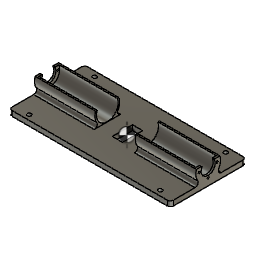
Bottenplatta v15 (Autodesk Fusion 360 design; units mm, degrees)
Autodesk Fusion 360 part; units mm, degrees
note: some values were not read from the file. Chosen so that the rebuilt part matches the saved one: add or cut; which face or edge a step refers to; which sketch regions a step uses.
sketch "Sketch1" plane through (0, 0, 0) normal (0, 0, 1) x (1, 0, 0)
  line L0 (-47, 8.9127) -> (107, 8.9127)
  line L1 (110, 11.9127) -> (110, 80.9127)
  line L2 (107, 83.9127) -> (-47, 83.9127)
  line L3 (-50, 80.9127) -> (-50, 11.9127)
  circle A0 centre (-35, 78.9127) radius 2
  line L4 (-70.7601, 46.4127) -> (89.2399, 46.4127)
  line L5 (30, -13.009) -> (30, 54.6952)
  circle A1 centre (95, 78.9127) radius 2
  circle A2 centre (-35, 13.9127) radius 2
  circle A3 centre (95, 13.9127) radius 2
  arc A4 (-47, 83.9127) -> (-50, 80.9127) centre (-47, 80.9127) ccw
  arc A5 (110, 80.9127) -> (107, 83.9127) centre (107, 80.9127) ccw
  arc A6 (107, 8.9127) -> (110, 11.9127) centre (107, 11.9127) ccw
  arc A7 (-50, 11.9127) -> (-47, 8.9127) centre (-47, 11.9127) ccw
  line L6 (35, 36.4127) -> (25, 36.4127)
  line L7 (25, 36.4127) -> (25, 56.4127)
  line L8 (25, 56.4127) -> (35, 56.4127)
  line L9 (35, 56.4127) -> (35, 36.4127)
  point P0 (110, 8.9127)
  point P1 (110, 83.9127)
  point P2 (-50, 83.9127)
  dimension "d3" = 4
  dimension "d4" = 15
  dimension "d5" = 5
  dimension "d6" = 75
  dimension "d7" = 160
  dimension "d9" = 75
  dimension "d12" = 3
  dimension "d13" = 160
  dimension "d48" = 50
  dimension "d57" = 20
  dimension "d58" = 10
  dimension "d59" = 27.5
  dimension "d60" = 75
  constraint horizontal L0
  constraint vertical L1
  constraint horizontal L2
  constraint vertical L3
  constraint perpendicular L1 L4
  constraint perpendicular L2 L5
  constraint symmetric A0 L5 A1
  constraint symmetric A0 L4 A2
  constraint symmetric L4 A1 A3
  constraint coincident P2 L2
  constraint coincident P2 L3
  constraint tangent L2 A4
  constraint tangent L3 A4
  constraint coincident P1 L1
  constraint coincident P1 L2
  constraint tangent L1 A5
  constraint tangent L2 A5
  constraint equal A4 A5
  constraint coincident P0 L0
  constraint coincident P0 L1
  constraint tangent L0 A6
  constraint tangent L1 A6
  constraint equal A4 A6
  constraint tangent L0 A7
  constraint tangent L3 A7
  constraint equal A4 A7
  constraint horizontal L6
  constraint vertical L7
  constraint horizontal L8
  constraint vertical L9
  measures "d3" diameter of A0
  measures "d4" distance of L3 A0.centre
  measures "d5" distance of L2 A0.centre
  measures "d6" distance of P0 P1
  measures "d7" distance of P1 P2
  measures "d12" radius of A4
  measures "d48" distance of origin L3
  measures "d57" distance of L6.start L8.end
  measures "d58" distance of L6.start L6.end
  measures "d59" distance of L0 L6
  measures "d60" distance of L1 L9
extrude "Extrude1" add sketch "Sketch1" along normal blind 3 contours L0 L3 L4 L5 A7 L6 L7 | L0 L1 L2 L3 L4 L5 A4 A5 A6 L6 L7 L8 L9
sketch "Sketch2" plane through (0, 0, 0) normal (0, 0, -1) x (1, 0, 0)
  circle A0 centre (95, -78.9127) radius 2
  circle A1 centre (-35, -13.9127) radius 2
  circle A2 centre (95, -13.9127) radius 2
  circle A3 centre (-35, -78.9127) radius 2
  arc A4 (-47, -8.9127) -> (-50, -11.9127) centre (-47, -11.9127) ccw
  line L0 (-50, -11.9127) -> (-50, -80.9127)
  arc A5 (-50, -80.9127) -> (-47, -83.9127) centre (-47, -80.9127) ccw
  line L1 (-47, -83.9127) -> (107, -83.9127)
  arc A6 (107, -83.9127) -> (110, -80.9127) centre (107, -80.9127) ccw
  line L2 (110, -80.9127) -> (110, -11.9127)
  arc A7 (110, -11.9127) -> (107, -8.9127) centre (107, -11.9127) ccw
  line L3 (107, -8.9127) -> (-47, -8.9127)
  line L4 (35, -56.4127) -> (25, -56.4127)
  line L5 (25, -56.4127) -> (25, -36.4127)
  line L6 (25, -36.4127) -> (35, -36.4127)
  line L7 (35, -36.4127) -> (35, -56.4127)
sketch "Sketch3" plane through (-50, 0, 0) normal (-1, 0, 0) x (0, -1, 0)
  line L0 (-80.9127, 0) -> (-11.9127, 0)
  line L1 (-11.9127, 0) -> (-11.9127, 3)
  line L2 (-11.9127, 3) -> (-80.9127, 3)
  line L3 (-80.9127, 3) -> (-80.9127, 0)
  circle A0 centre (-46.4127, 14) radius 10.8
  line L4 (-11.9127, 0) -> (-80.9127, 0)
  circle A1 centre (-46.4127, 14) radius 12.3
  line L5 (-33, 21) -> (-5, 21)
  line L6 (-83.9127, 0) -> (-83.9127, 3)
  line L7 (-8.9127, 0) -> (-8.9127, 3)
  dimension "d14" = 21.6
  dimension "d15" = 14
  dimension "d16" = 1.5
  dimension "d33" = 75
  dimension "d34" = 37.5
  constraint horizontal L5
  measures "d14" diameter of A0
  measures "d15" distance of A0.centre L4
  measures "d33" distance of L6 L7
  measures "d34" distance of A0.centre L7
sketch "Sketch4" plane through (110, 0, 0) normal (1, 0, 0) x (0, 1, 0)
  line L0 (11.9127, 0) -> (80.9127, 0)
  line L1 (80.9127, 0) -> (80.9127, 3)
  line L2 (80.9127, 3) -> (11.9127, 3)
  line L3 (11.9127, 3) -> (11.9127, 0)
  circle A0 centre (46.4127, 14) radius 10.8
  line L4 (33, 21) -> (5, 21)
  circle A1 centre (46.4127, 14) radius 12.3
extrude "Extrude2" add sketch "Sketch4" against normal blind 60 contours L2 A1 picked at (35.797, 8.8983)
extrude "Extrude3" add sketch "Sketch3" against normal blind 60 contours L2 A1 picked at (-57.0284, 8.8983)
sketch "Sketch5" plane through (110, 0, 0) normal (1, 0, 0) x (0, 1, 0)
  circle A0 centre (46.4127, 14) radius 10.8
  line L0 (11.9127, 0) -> (80.9127, 0)
  line L1 (80.9127, 0) -> (80.9127, 3)
  line L2 (80.9127, 3) -> (51.9163, 3)
  arc A1 (51.9163, 3) -> (40.9091, 3) centre (46.4127, 14) ccw
  line L3 (40.9091, 3) -> (11.9127, 3)
  line L4 (11.9127, 3) -> (11.9127, 0)
  circle A2 centre (37.4127, 14) radius 1
  circle A3 centre (46.4127, 5) radius 1
  circle A4 centre (55.4127, 14) radius 1
  circle A5 centre (46.4127, 23) radius 1
  dimension "d23" = 2
  dimension "d24" = 9
  dimension "d26" = 360
  constraint horizontal A2.centre A4.centre
  measures "d23" diameter of A2
  measures "d24" distance of A0.centre A2.centre
extrude "Extrude4" add sketch "Sketch5" against normal blind 2 contours A0 | L0 L1 L2 A1 L3 L4
sketch "Sketch6" plane through (110, 0, 0) normal (1, 0, 0) x (0, 1, 0)
  circle A0 centre (37.4127, 14) radius 1
  circle A1 centre (46.4127, 5) radius 1
  circle A2 centre (55.4127, 14) radius 1
  circle A3 centre (46.4127, 23) radius 1
  line L0 (11.9127, 0) -> (80.9127, 0)
  line L1 (80.9127, 0) -> (80.9127, 3)
  line L2 (80.9127, 3) -> (51.9163, 3)
  arc A4 (51.9163, 3) -> (40.9091, 3) centre (46.4127, 14) ccw
  line L3 (40.9091, 3) -> (11.9127, 3)
  line L4 (11.9127, 3) -> (11.9127, 0)
  circle A5 centre (46.4127, 14) radius 7
  line L5 (46.4127, 14) -> (53.2094, 20.7967)
  line L6 (46.4127, 14) -> (51.6312, 14) construction
  dimension "d29" = 14
  dimension "d42" = 45
  constraint concentric A4 A5
  constraint horizontal L6
  constraint coincident A4.centre A5.centre
  measures "d29" diameter of A5
  measures "d42" angle of L5 L6
extrude "Extrude5" cut sketch "Sketch6" against normal blind 2 contours A5
sketch "Sketch7" plane through (-50, 0, 0) normal (-1, 0, 0) x (0, -1, 0)
  circle A0 centre (-46.4127, 14) radius 10.8
  line L0 (-80.9127, 0) -> (-11.9127, 0)
  line L1 (-11.9127, 0) -> (-11.9127, 3)
  line L2 (-11.9127, 3) -> (-40.9091, 3)
  arc A1 (-40.9091, 3) -> (-51.9163, 3) centre (-46.4127, 14) ccw
  line L3 (-51.9163, 3) -> (-80.9127, 3)
  line L4 (-80.9127, 3) -> (-80.9127, 0)
  line L5 (-70, 18) -> (-12.2133, 18)
  dimension "d37" = 15
  constraint horizontal L5
  measures "d37" distance of L2 L5
extrude "Extrude6" cut sketch "Sketch7" against normal through all contours A0 L5 | A0 A1 L5 picked at (-48.2013, 22.18)
fillet "Fillet2" radius 3 6 edges at (80, 40.9091, 3) (-20, 51.9163, 3) (-20, 51.9163, 3) (-20, 40.9091, 3) (80, 40.9091, 3) (80, 51.9163, 3)
sketch "Sketch8" plane through (-50, 0, 0) normal (-1, 0, 0) x (0, -1, 0)
  line L0 (-34.7813, 18) -> (-36.3808, 18)
  arc A0 (-56.4447, 18) -> (-36.3808, 18) centre (-46.4127, 14) ccw
  line L1 (-56.4447, 18) -> (-58.0441, 18)
  arc A1 (-58.0441, 18) -> (-56.8973, 7.5686) centre (-46.4127, 14) ccw
  arc A2 (-59.4546, 3) -> (-56.8973, 7.5686) centre (-59.4546, 6) ccw
  line L2 (-59.4546, 3) -> (-80.9127, 3)
  line L3 (-80.9127, 3) -> (-80.9127, 0)
  line L4 (-80.9127, 0) -> (-11.9127, 0)
  line L5 (-11.9127, 0) -> (-11.9127, 3)
  line L6 (-11.9127, 3) -> (-33.3709, 3)
  arc A3 (-35.9281, 7.5686) -> (-33.3709, 3) centre (-33.3709, 6) ccw
  arc A4 (-35.9281, 7.5686) -> (-34.7813, 18) centre (-46.4127, 14) ccw
  circle A5 centre (-37.4127, 14) radius 1
  circle A6 centre (-46.4127, 5) radius 1
  circle A7 centre (-55.4127, 14) radius 1
  line L7 (-36.3808, 18) -> (-40.6681, 18)
  arc A8 (-52.1573, 18) -> (-40.6681, 18) centre (-46.4127, 14) ccw
  line L8 (-52.1573, 18) -> (-56.4447, 18)
  arc A9 (-56.4447, 18) -> (-36.3808, 18) centre (-46.4127, 14) ccw
extrude "Extrude7" cut sketch "Sketch8" against normal blind 2 contours A0 L7 A8 L8 A9
fillet "Fillet3" radius 0.5 2 edges at (109, 52.1573, 18) (109, 40.6681, 18)
extrude "Extrude8" add sketch "Sketch8" against normal blind 2
fillet "Fillet4" radius 0.5 2 edges at (-49, 40.6681, 18) (-49, 52.1573, 18)
extrude "Extrude9" add sketch "Sketch2" along normal blind 2
equation "d9 = d6"
equation "d13 = d7"
equation "d34 = d33 / 2"
equation "d59 = ( d6 - d57 ) / 2"
equation "d60 = ( d13 - d58 ) / 2"
named bodies: "Bottenplatta"
